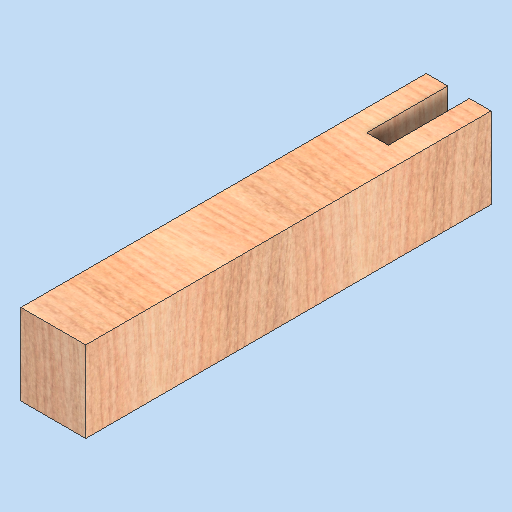
# Autodesk Inventor part: SeatBeam100x80
Saved by Autodesk Inventor 2023 (Build 270158000, 158)
## iProperties
Created: 2026-03-22
Part Number: SeatBeam100x80
Material: Wood (Birch)
Document SubType Name: Modeling
Designer: Nathann
Density: 0.55 g/cm^3
Appearance: Birch - Natural Polished
Mass: 2053.33 g
Surface Area: 2106.67 cm^2
Volume: 3733.33 cm^3
Author: Nathann
Autodesk Inventor part; units mm, degrees
ref_plane "YZ Plane" through (0, 0, 0) normal (1, 0, 0) x (0, 1, 0)
ref_plane "XZ Plane" through (0, 0, 0) normal (0, 1, 0) x (-1, 0, 0)
ref_plane "XY Plane" through (0, 0, 0) normal (0, 0, 1) x (1, 0, 0)
sketch "Sketch1" plane through (0, 0, 0) normal (0, 1, 0) x (-1, 0, 0)
  line L0 (26.6667, 0) -> (53.3333, 0)
  line L1 (80, 0) -> (80, 400)
  line L2 (80, 400) -> (0, 400)
  line L3 (0, 400) -> (0, 0)
  line L4 (80, 0) -> (53.3333, 0)
  line L5 (53.3333, 0) -> (53.3333, -100)
  line L6 (53.3333, -100) -> (80, -100)
  line L7 (80, -100) -> (80, 0)
  line L8 (0, 0) -> (26.6667, 0)
  line L9 (26.6667, 0) -> (26.6667, -100)
  line L10 (26.6667, -100) -> (0, -100)
  line L11 (0, -100) -> (0, 0)
  dimension "d0" = 80
  dimension "d1" = 400
  dimension "d2" = 100
  dimension "d3" = 100
  dimension "d4" = 26.6667
  dimension "d5" = 26.6667
  constraints: 24 end point, 6 parallel, 3 horizontal, 3 perpendicular
  measures "d0" distance of L1.end L2.end
  measures "d1" distance of L1.start L1.end
  measures "d2" distance of L6.end L1.start
  measures "d3" distance of L10.end L3.end
  measures "d4" distance of L5.end L6.end
  measures "d5" distance of L9.end L10.end
extrude "Extrusion1" add sketch "Sketch1" along normal blind 100
equation "\"d5\" = d4"
body "Solid1"
